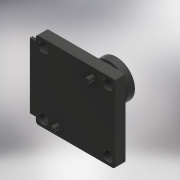
# Autodesk Inventor part: xtion_rgb_cam
Saved by Autodesk Inventor 2017 (Build 210142000, 142)
## iProperties
Created: 2016-11-18
Part Number: xtion_rgb_cam
Material: Thermoplastic Resin
Document SubType Name: Modeling
Designer: Ali
Density: 1.28 g/cm^3
Appearance: Smooth - Black
Author: Ali
Autodesk Inventor part; units mm, degrees
ref_plane "YZ Plane" through (0, 0, 0) normal (1, 0, 0) x (0, 1, 0)
ref_plane "XZ Plane" through (0, 0, 0) normal (0, 1, 0) x (-1, 0, 0)
ref_plane "XY Plane" through (0, 0, 0) normal (0, 0, 1) x (1, 0, 0)
sketch "Sketch1" plane through (0, 0, 0) normal (0, 1, 0) x (-1, 0, 0)
  line L0 (-8, 7.8) -> (8, 7.8)
  line L1 (8, 7.8) -> (8, -7.8)
  line L2 (8, -7.8) -> (-8, -7.8)
  line L3 (-8, -7.8) -> (-8, 7.8)
  line L4 (-8, 7.8) -> (8, -7.8) construction
  line L5 (8, 7.8) -> (-8, -7.8) construction
  point P0 (0, 0)
  dimension "d0" = 16
  dimension "d1" = 15.6
  constraints: 12 end point, 2 midpoint, 2 parallel, 1 horizontal, 1 perpendicular
  measures "d0" distance of L1.end L2.end
  measures "d1" distance of L0.end L1.end
extrude "Extrusion1" add sketch "Sketch1" along normal blind 2.1
sketch "Sketch2" plane through (0, 0, 0) normal (0, -1, 0) x (1, 0, 0)
  circle A0 centre (3.5, 6) radius 0.5
  circle A1 centre (-3.5, -6) radius 0.5
  line L0 (-3.5, -6) -> (3.5, 6) construction
  point P0 (0, 0)
  point P1 (0, 0)
  dimension "d4" = 1
  dimension "d5" = 1
  dimension "d6" = 12
  dimension "d7" = 7
  constraints: 2 centre point, 2 end point, 1 coincident, 1 midpoint
  measures "d4" diameter of A0
  measures "d5" diameter of A1
  measures "d6" vertical distance of L0.start L0.end
  measures "d7" horizontal distance of L0.end L0.start
extrude "Extrusion2" add sketch "Sketch2" along normal blind 1.2
sketch "Sketch3" plane through (0, 2.1, 0) normal (0, 1, 0) x (1, 0, 0)
  line L0 (-6.5, -6.25) -> (6.5, -6.25)
  line L1 (6.5, -6.25) -> (6.5, 6.25)
  line L2 (6.5, 6.25) -> (-6.5, 6.25)
  line L3 (-6.5, 6.25) -> (-6.5, -6.25)
  line L4 (-6.5, -6.25) -> (6.5, 6.25) construction
  line L5 (6.5, -6.25) -> (-6.5, 6.25) construction
  point P0 (0, 0)
  dimension "d10" = 13
  dimension "d11" = 12.5
  constraints: 12 end point, 4 coincident, 2 midpoint, 2 parallel, 1 horizontal, 1 perpendicular
  measures "d10" distance of L2.end L1.end
  measures "d11" distance of L1.end L0.end
hole "Hole1" at (-6.5, 2.1, -6.25) at (6.5, 2.1, -6.25) at (6.5, 2.1, 6.25) at (-6.5, 2.1, 6.25) direction (0, -1, 0) diameter 2 end through all
sketch "Sketch4" plane through (0, 0, 0) normal (0, 0, 1) x (1, 0, 0)
  line L0 (8, 0) -> (-8, 0) projected
  line L1 (8, 0) -> (8, 2.1) projected
  line L2 (-8, 2.1) -> (8, 2.1) projected
  line L3 (-8, 0) -> (-8, 2.1) projected
  line L4 (-8, 2.1) -> (8, 2.1) projected
  line L5 (0, 2.1) -> (0, 21.9)
  line L6 (4.5, 2.1) -> (4.5, 4.7)
  line L7 (4.5, 4.7) -> (3.25, 4.7)
  line L8 (3.25, 4.7) -> (3.25, 6.76)
  line L9 (3.25, 6.76) -> (3.75, 6.76)
  line L10 (3.75, 6.76) -> (3.75, 8.26)
  line L11 (3.75, 8.26) -> (2.95, 8.26)
  line L12 (2.95, 8.26) -> (2.7737, 7.26)
  line L13 (2.7737, 7.26) -> (2, 6.8133)
  line L14 (2, 6.8133) -> (2, 6.5468)
  arc A0 (2, 6.5468) -> (0, 7.7678) centre (0, 5.5193) ccw
  point P0 (0, 0)
  dimension "d19" = 9
  dimension "d20" = 6.5
  dimension "d21" = 7.5
  dimension "d22" = 0.8
  dimension "d23" = 1
  dimension "d24" = 80
  dimension "d25" = 120
  dimension "d26" = 2.6
  dimension "d27" = 2.06
  dimension "d28" = 1.5
  dimension "d29" = 1.25
  constraints: 20 end point, 5 perpendicular, 3 point on line, 3 vertical, 2 point on circle, 1 centre point, 1 midpoint
  measures "d19" diameter of L6 L5
  measures "d20" diameter of L8 L5
  measures "d21" diameter of L10 L5
  measures "d22" distance of L10.end L11.end
  measures "d23" distance from line of L11 L12.end
  measures "d24" angle of L12 L11
  measures "d25" angle of L13 L10
  measures "d26" distance of L6.start L6.end
  measures "d27" distance of L7.end L8.end
  measures "d28" distance of L9.end L10.end
  measures "d29" distance between parallel lines of L8 L14
revolve "Revolution1" add sketch "Sketch4" angle 360 about axis through (0, 2.1, 0) along (0, 1, 0) contours L2 L5 A0 L14 L13 L12 L11 L10 L9 L8 L7 L6
fillet "Fillet1" radius 0.5 4 edges at (-8, 1.05, 7.8) (-8, 1.05, -7.8) (8, 1.05, -7.8) (8, 1.05, 7.8)
sketch "Sketch5" plane through (-8, 0, -7.3) normal (-1, 0, 0) x (0, 0, 1)
  line L0 (0.7033, 0.536) -> (13.8967, 0.536)
  line L1 (13.8967, 0.536) -> (13.8967, 0)
  line L2 (13.8967, 0) -> (0.7033, 0)
  line L3 (0.7033, 0) -> (0.7033, 0.536)
  line L4 (0.7033, 0.536) -> (13.8967, 0) construction
  line L5 (13.8967, 0.536) -> (0.7033, 0) construction
  line L6 (14.6, 0) -> (0, 0) projected
  point P0 (7.3, 0)
  point P1 (7.3, 0.268)
  point P2 (7.3, 0)
  constraints: 12 end point, 4 midpoint, 2 parallel, 1 horizontal, 1 perpendicular
extrude "Extrusion3" add sketch "Sketch5" along normal blind 1.2
body "Solid1"
